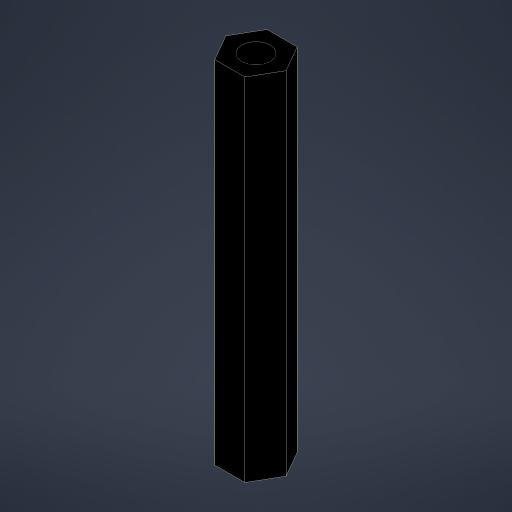
# Autodesk Inventor part: Standoff_M3_37mm
Saved by Autodesk Inventor 2025 (Build 290162010, 162A)
## iProperties
Created: 2023-06-26
Part Number: Standoff_M3_37mm
Material: Aluminum 6061
Document SubType Name: Modeling
Designer: dzw04
Density: 2.7 g/cm^3
Appearance: Anodized - Black
Author: dzw04
Autodesk Inventor part; units mm, degrees
ref_plane "YZ Plane" through (0, 0, 0) normal (1, 0, 0) x (0, 1, 0)
ref_plane "XZ Plane" through (0, 0, 0) normal (0, 1, 0) x (-1, 0, 0)
ref_plane "XY Plane" through (0, 0, 0) normal (0, 0, 1) x (1, 0, 0)
sketch "Sketch1" plane through (0, 0, 0) normal (0, 1, 0) x (-1, 0, 0)
  line L0 (3.1754, 0) -> (1.5877, -2.75)
  line L1 (1.5877, -2.75) -> (-1.5877, -2.75)
  line L2 (-1.5877, -2.75) -> (-3.1754, 0)
  line L3 (-3.1754, 0) -> (-1.5877, 2.75)
  line L4 (-1.5877, 2.75) -> (1.5877, 2.75)
  line L5 (1.5877, 2.75) -> (3.1754, 0)
  circle A0 centre (0, 0) radius 1.5
  dimension "d0" = 5.5
  dimension "d1" = 3
  constraints: 12 end point, 2 coincident, 1 centre point, 1 horizontal, 13 other
  measures "d0" distance between parallel lines of L1 L4
  measures "d1" diameter of A0
extrude "Extrusion1" add sketch "Sketch1" along normal blind 37
body "Solid1"
